Autodesk Inventor part; units mm, degrees
(part 2 of 2)
  line L319 (-28.6263, 18.3241) -> (-28.6263, 16.0044)
  line L320 (-28.6263, 16.0044) -> (-25.6449, 16.0044)
  line L321 (-25.6449, 18.3241) -> (-28.6263, 18.3241)
  line L322 (-29.7503, 19.4482) -> (-24.5209, 19.4482)
  line L323 (-29.5884, 13.8513) -> (-27.9357, 13.8513)
  line L324 (-29.5884, 12.8808) -> (-29.5884, 13.8513)
  line L325 (-29.7503, 14.8804) -> (-29.7503, 19.4482)
  line L326 (-26.6942, 13.8513) -> (-19.7097, 13.8513)
  line L327 (-23.8, 11.9101) -> (-23.8, 12.8808)
  line L328 (-25.8364, 11.9101) -> (-23.8, 11.9101)
  line L329 (-24.7124, 10.786) -> (-24.7124, 8.4664)
  line L330 (-21.731, 8.4664) -> (-21.731, 10.786)
  line L331 (-24.7124, 8.4664) -> (-21.731, 8.4664)
  line L332 (-21.731, 10.786) -> (-24.7124, 10.786)
  line L333 (-26.6942, 14.8804) -> (-26.6942, 13.8513)
  line L334 (-24.5209, 14.8804) -> (-26.6942, 14.8804)
  line L335 (-20.607, 11.9101) -> (-20.607, 7.3423)
  line L336 (-20.607, 7.3423) -> (-25.8364, 7.3423)
  line L337 (-25.8364, 7.3423) -> (-25.8364, 11.9101)
  line L338 (-27.9357, 14.8804) -> (-29.7503, 14.8804)
  line L339 (-50.2795, 78.7871) -> (-51.4898, 78.7871)
  line L340 (-51.4898, 78.7871) -> (-51.4898, 75.2962)
  line L341 (-51.4898, 75.2962) -> (-52.7989, 75.2962)
  line L342 (-52.7989, 75.2962) -> (-52.7989, 78.7871)
  line L343 (-52.7989, 78.7871) -> (-57.2861, 78.7871)
  line L344 (-57.2861, 78.7871) -> (-57.2861, 80.2197)
  line L345 (-57.2861, 80.2197) -> (-52.7413, 85.4562)
  line L346 (-52.7413, 85.4562) -> (-51.4898, 85.4562)
  line L347 (-51.4898, 85.4562) -> (-51.4898, 79.8822)
  line L348 (-51.4898, 79.8822) -> (-50.2795, 79.8822)
  line L349 (-50.2795, 79.8822) -> (-50.2795, 78.7871)
  line L350 (-52.7989, 79.8822) -> (-52.7989, 83.8507)
  line L351 (-52.7989, 83.8507) -> (-56.2158, 79.8822)
  line L352 (-56.2158, 79.8822) -> (-52.7989, 79.8822)
  line L353 (-13.2205, 10.2825) -> (-12.0102, 10.2825)
  line L354 (-12.0102, 10.2825) -> (-12.0102, 13.7735)
  line L355 (-12.0102, 13.7735) -> (-10.7011, 13.7735)
  line L356 (-10.7011, 13.7735) -> (-10.7011, 10.2825)
  line L357 (-10.7011, 10.2825) -> (-6.2139, 10.2825)
  line L358 (-6.2139, 10.2825) -> (-6.2139, 8.8499)
  line L359 (-6.2139, 8.8499) -> (-10.7587, 3.6135)
  line L360 (-10.7587, 3.6135) -> (-12.0102, 3.6135)
  line L361 (-12.0102, 3.6135) -> (-12.0102, 9.1875)
  line L362 (-12.0102, 9.1875) -> (-13.2205, 9.1875)
  line L363 (-13.2205, 9.1875) -> (-13.2205, 10.2825)
  line L364 (-10.7011, 9.1875) -> (-10.7011, 5.219)
  line L365 (-10.7011, 5.219) -> (-7.2842, 9.1875)
  line L366 (-7.2842, 9.1875) -> (-10.7011, 9.1875)
  line L367 (-13.2205, 10.2825) -> (-12.0102, 10.2825)
  line L368 (-12.0102, 10.2825) -> (-12.0102, 13.7735)
  line L369 (-12.0102, 13.7735) -> (-10.7011, 13.7735)
  line L370 (-10.7011, 13.7735) -> (-10.7011, 10.2825)
  line L371 (-10.7011, 10.2825) -> (-6.2139, 10.2825)
  line L372 (-6.2139, 10.2825) -> (-6.2139, 8.8499)
  line L373 (-6.2139, 8.8499) -> (-10.7587, 3.6135)
  line L374 (-10.7587, 3.6135) -> (-12.0102, 3.6135)
  line L375 (-12.0102, 3.6135) -> (-12.0102, 9.1875)
  line L376 (-12.0102, 9.1875) -> (-13.2205, 9.1875)
  line L377 (-13.2205, 9.1875) -> (-13.2205, 10.2825)
  line L378 (-10.7011, 9.1875) -> (-10.7011, 5.219)
  line L379 (-10.7011, 5.219) -> (-7.2842, 9.1875)
  line L380 (-7.2842, 9.1875) -> (-10.7011, 9.1875)
  line L381 (-50.2795, 78.7871) -> (-51.4898, 78.7871)
  line L382 (-51.4898, 78.7871) -> (-51.4898, 75.2962)
  line L383 (-51.4898, 75.2962) -> (-52.7989, 75.2962)
  line L384 (-52.7989, 75.2962) -> (-52.7989, 78.7871)
  line L385 (-52.7989, 78.7871) -> (-57.2861, 78.7871)
  line L386 (-57.2861, 78.7871) -> (-57.2861, 80.2197)
  line L387 (-57.2861, 80.2197) -> (-52.7413, 85.4562)
  line L388 (-52.7413, 85.4562) -> (-51.4898, 85.4562)
  line L389 (-51.4898, 85.4562) -> (-51.4898, 79.8822)
  line L390 (-51.4898, 79.8822) -> (-50.2795, 79.8822)
  line L391 (-50.2795, 79.8822) -> (-50.2795, 78.7871)
  line L392 (-52.7989, 79.8822) -> (-52.7989, 83.8507)
  line L393 (-52.7989, 83.8507) -> (-56.2158, 79.8822)
  line L394 (-56.2158, 79.8822) -> (-52.7989, 79.8822)
  point P0 (-40.5846, 75.534)
  point P1 (-53.7479, 68.8958)
  point P2 (-9.7521, 20.0042)
  point P3 (-41.8348, 101.4209)
  point P4 (-40.5846, 75.534)
  point P5 (-53.7479, 68.8958)
  point P6 (-9.7521, 20.0042)
  point P7 (-1, 6.9835)
  point P8 (-22.9154, 75.534)
  point P9 (-94.7005, 61.8998)
  point P10 (-94.7005, 61.8998)
  point P11 (-22.9154, 75.534)
  point P12 (-22.9154, 75.534)
  point P13 (-40.5846, 13.366)
  point P14 (-22.9154, 13.366)
  point P15 (-40.5846, 13.366)
  point P16 (-40.5846, 13.366)
  point P17 (-22.9154, 13.366)
  point P18 (-22.9154, 13.366)
  dimension "d155" = 8.4153
  dimension "d157" = 0.508
  dimension "d158" = 4.5466
  dimension "d159" = 0.508
  dimension "d160" = 4.5466
  constraints: 652 end point, 50 parallel, 20 perpendicular, 14 horizontal, 5 midpoint, 1 symmetric about line, 14 other
  measures "d155" distance of L174.end L172.start
  measures "d157" distance between parallel lines of L7 L173
  measures "d158" distance from line of point (-1, 6.983) L172
  measures "d159" distance between parallel lines of L6 L168
  measures "d160" distance between parallel lines of L4 L171
extrude "Extrusion20" add sketch "Sketch17" along normal blind 0.4 contours L48 L49 L73 L71 L76 L69 L86 L79 L85 L67 L62 L68 L84 L80 L87 L77 L82 L60 L55 L61 L81 L78 L83 L70 L75 L72 L74 L50 | L88 L89 L113 L111 L116 L109 L126 L119 L125 L107 L102 L108 L124 L120 L127 L117 L122 L100 L95 L101 L121 L118 L123 L110 L115 L112 L114 L90 | L128 L129 L153 L151 L156 L149 L166 L159 L165 L147 L142 L148 L164 L160 L167 L157 L162 L140 L135 L141 L161 L158 L163 L150 L155 L152 L154 L130 | L219 L225 L226 L229 L230 L231 L234 L232 L233 L249 L247 L248 L257 L256 L237 L238 L239 L235 L246 L245 L244 L241 L255 L254 L258 L228 L223 L224 | L260 L272 L269 L268 L270 L277 L266 L274 L276 L295 L296 L297 L288 L287 L263 L284 L283 L273 L298 L285 L282 L278 L294 L293 L286 L267 L264 L275 | L300 L312 L309 L308 L310 L317 L306 L314 L316 L335 L336 L337 L328 L327 L303 L324 L323 L313 L338 L325 L322 L318 L334 L333 L326 L307 L304 L315 | L339 L340 L341 L342 L343 L344 L345 L346 L347 L348 L349 | L353 L354 L355 L356 L357 L358 L359 L360 L361 L362 L363 bodies 2
sketch "Sketch18" plane through (0, 0, -0.2) normal (0, 0, -1) x (-1, 0, 0)
  line L0 (0, 0) -> (-63.5, 0)
  line L1 (-63.5, 0) -> (-63.5, 88.9)
  line L2 (-63.5, 88.9) -> (0, 88.9)
  line L3 (0, 88.9) -> (0, 0)
  constraints: 8 end point, 2 parallel, 1 horizontal, 1 perpendicular
extrude "Extrusion21" add sketch "Sketch18" along normal blind 0.4 bodies 3
fillet "Fillet2" radius 3.175 8 edges at (63.5, 0, 0.2) (63.5, 88.9, 0.2) (0, 0, 0.2) (0, 88.9, 0.2) (63.5, 0, -0.3) (63.5, 88.9, -0.3) (0, 0, -0.3) (0, 88.9, -0.3)
extrude "Extrusion22" cut sketch "Sketch17" along normal blind 0.4 contours L48 L49 L73 L71 L76 L69 L86 L79 L85 L67 L62 L68 L84 L80 L87 L77 L82 L60 L55 L61 L81 L78 L83 L70 L75 L72 L74 L50 | L88 L89 L113 L111 L116 L109 L126 L119 L125 L107 L102 L108 L124 L120 L127 L117 L122 L100 L95 L101 L121 L118 L123 L110 L115 L112 L114 L90 | L128 L129 L153 L151 L156 L149 L166 L159 L165 L147 L142 L148 L164 L160 L167 L157 L162 L140 L135 L141 L161 L158 L163 L150 L155 L152 L154 L130 | L219 L225 L226 L229 L230 L231 L234 L232 L233 L249 L247 L248 L257 L256 L237 L238 L239 L235 L246 L245 L244 L241 L255 L254 L258 L228 L223 L224 | L260 L272 L269 L268 L270 L277 L266 L274 L276 L295 L296 L297 L288 L287 L263 L284 L283 L273 L298 L285 L282 L278 L294 L293 L286 L267 L264 L275 | L300 L312 L309 L308 L310 L317 L306 L314 L316 L335 L336 L337 L328 L327 L303 L324 L323 L313 L338 L325 L322 L318 L334 L333 L326 L307 L304 L315 | L339 L340 L341 L342 L343 L344 L345 L346 L347 L348 L349 | L353 L354 L355 L356 L357 L358 L359 L360 L361 L362 L363 bodies 3
